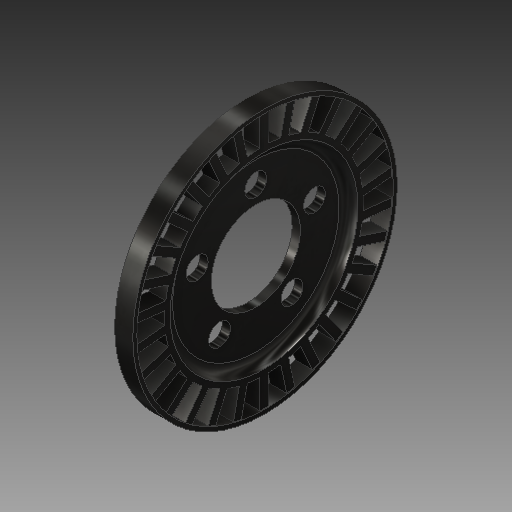
# Autodesk Inventor part: 362-10
Saved by Autodesk Inventor 2019 (Build 230136000, 136)
## iProperties
Company: Autodesk Inc.
Created: 2017-03-19
Part Number: 362-10
Material: Titanium
Document SubType Name: Modeling
Designer: Autodesk Inc.
Density: 4.51 g/cm^3
Appearance: Anodized - Subtle Dark Bronze Satin
Mass: 712.012 g
Surface Area: 715.037 cm^2
Volume: 157.874 cm^3
Author: Inventor
Autodesk Inventor part; units mm, degrees
ref_plane "YZ Plane" through (0, 0, 0) normal (1, 0, 0) x (0, 1, 0)
ref_plane "XZ Plane" through (0, 0, 0) normal (0, 1, 0) x (-1, 0, 0)
sketch "Sketch1" plane through (0, 0, 0) normal (1, 0, 0) x (0, 1, 0)
  circle A0 centre (0, 0) radius 32.5
  circle A1 centre (0, 0) radius 72.5
  dimension "d1" = 65
  dimension "d2" = 145
  constraints: 2 centre point, 1 coincident
  measures "d1" diameter of A0
  measures "d2" diameter of A1
extrude "Extrusion1" add sketch "Sketch1" along normal blind 12
sketch "Sketch2" plane through (12, 0, 0) normal (1, 0, 0) x (0, 0, -1)
  circle A0 centre (0, 0) radius 68.5
  dimension "d17" = 137
  constraints: 1 centre point, 1 coincident
  measures "d17" diameter of A0
extrude "Extrusion2" cut sketch "Sketch2" against normal blind 6
ref_plane "Work Plane1" through (-0.5, 0, 0) normal (-1, 0, 0) x (0, 0, 1)
sketch "Sketch4" plane through (-0.5, 0, 0) normal (-1, 0, 0) x (0, 0, 1)
  circle A0 centre (0, 0) radius 96.5
  circle A1 centre (0, 0) radius 93.5
  dimension "d21" = 193
  dimension "d22" = 187
  constraints: 2 centre point, 2 coincident
  measures "d21" diameter of A0
  measures "d22" diameter of A1
extrude "Extrusion3" add sketch "Sketch4" against normal blind 13.228
sketch "Sketch5" plane through (0, 0, 0) normal (-1, 0, 0) x (0, 0, 1)
  line L0 (0, -127.8255) -> (0, 105.8876) construction
  line L1 (-101.5, 0) -> (101.5, 0) construction
  line L2 (3, -94.4379) -> (-3, -94.4379)
  line L3 (-3, -94.4379) -> (-3, -72.4379)
  line L4 (-3, -72.4379) -> (3, -72.4379)
  line L5 (3, -72.4379) -> (3, -94.4379)
  circle A0 centre (0, 0) radius 72.5 construction
  point P0 (0, 0)
  point P1 (0, -72.4379)
  dimension "d26" = 6
  dimension "d27" = 22
  constraints: 8 end point, 2 parallel, 1 horizontal, 1 midpoint, 1 perpendicular, 1 point on line, 2 other
  measures "d26" distance of L3.end L4.end
  measures "d27" distance of L2.end L3.end
extrude "Extrusion4" add sketch "Sketch5" against normal up to surface (12 mm away)
pattern_circular "Circular Pattern1" count 30 over 360 about axis through (-10, 0, 0) along (1, 0, 0) of "Extrusion4"
fillet "Fillet3" radius 8 1 edges at (6, 0, 68.5)
sketch "Sketch6" plane through (0, 72.4379, 3) normal (-1, 0, 0) x (0, 0, 1)
  circle A0 centre (-3, -72.4379) radius 45 construction
  line L0 (-3, -74.5336) -> (-3, -4.9042) construction
  circle A1 centre (-3, -27.4379) radius 8
  circle A2 centre (-3, -72.4379) radius 93.5 projected
  dimension "d37" = 90
  dimension "d40" = 16
  constraints: 2 end point, 2 vertical alignment, 1 centre point, 1 coincident, 1 point on line, 1 vertical, 2 other
  measures "d40" diameter of A1
extrude "Extrusion5" cut sketch "Sketch6" against normal through all contours A1
pattern_circular "Circular Pattern2" count 5 over 360 about axis through (-10, 0, 0) along (1, 0, 0) of "Extrusion5"
sketch "Sketch7" plane through (6, 0, 0) normal (1, 0, 0) x (0, 0, -1)
  point P0 (0, 0)
body "Solid1"
